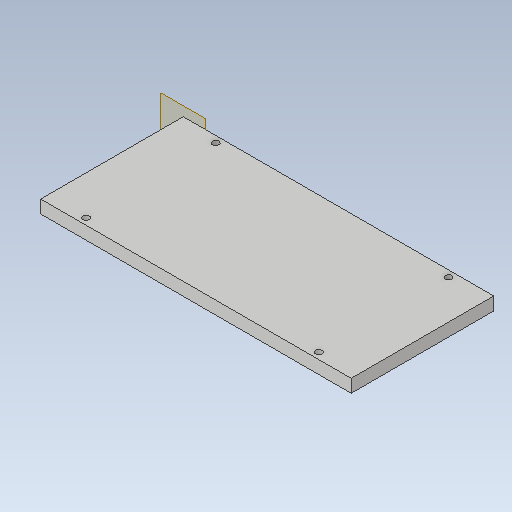
# Autodesk Inventor part: Base
Saved by Autodesk Inventor 2020 (Build 240168000, 168)
## iProperties
Created: 2020-04-07
Part Number: Base
Material: Generic
Document SubType Name: Modeling
Designer: gman
Density: 1 g/cm^3
Appearance: Default
Mass: 67.2716 g
Surface Area: 242.603 cm^2
Volume: 67.2716 cm^3
Author: gman
Autodesk Inventor part; units mm, degrees
ref_plane "YZ Plane" through (0, 0, 0) normal (1, 0, 0) x (0, 1, 0)
ref_plane "XZ Plane" through (0, 0, 0) normal (0, 1, 0) x (-1, 0, 0)
ref_plane "XY Plane" through (0, 0, 0) normal (0, 0, 1) x (1, 0, 0)
ref_plane "Work Plane1" through (0, 0, 152.1968) normal (0, 0, 1) x (1, 0, 0)
sketch "Sketch2" plane through (0, 0, 152.1968) normal (0, 0, 1) x (1, 0, 0)
  line L0 (0, 0) -> (152.1206, 0)
  line L1 (152.1206, 0) -> (152.1206, 6.35)
  line L2 (152.1206, 6.35) -> (0, 6.35)
  line L3 (0, 6.35) -> (0, 0)
  dimension "d20" = 152.1206
  dimension "d21" = 6.35
  constraints: 8 end point, 2 parallel, 1 horizontal, 1 perpendicular
  measures "d20" distance of L0.start L0.end
  measures "d21" distance of L0.end L1.end
extrude "Extrusion2" add sketch "Sketch2" along normal blind 69.85
sketch "Sketch4" plane through (0, 6.35, 152.1968) normal (0, 1, 0) x (1, 0, 0)
  circle A0 centre (19.05, -3.175) radius 1.5875
  circle A1 centre (133.0706, -3.175) radius 1.5875
  circle A2 centre (133.0706, -66.675) radius 1.5875
  circle A3 centre (19.05, -66.675) radius 1.5875
  line L0 (0, 0) -> (0, -69.85) projected
  line L1 (152.1206, 0) -> (0, 0) projected
  line L2 (152.1206, 0) -> (152.1206, -69.85) projected
  line L3 (152.1206, -69.85) -> (0, -69.85) projected
  point P0 (0, 152.1968)
  dimension "d22" = 3.175
  dimension "d23" = 19.05
  dimension "d24" = 3.175
  dimension "d25" = 19.05
  dimension "d26" = 3.175
  constraints: 4 centre point, 3 equal radius, 2 horizontal alignment, 2 vertical alignment
  measures "d22" diameter of A0
  measures "d23" distance from line of L0 A0.centre
  measures "d24" distance from line of L1 A0.centre
  measures "d25" distance from line of L2 A1.centre
  measures "d26" distance from line of L3 A2.centre
extrude "Extrusion4" cut sketch "Sketch4" against normal blind 152.1968 contours A0 | A1 | A2 | A3
body "Solid2"
